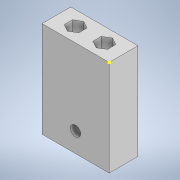
# Autodesk Inventor part: bumper piece 1
Saved by Autodesk Inventor 2022 (Build 260153000, 153)
## iProperties
Created: 2023-01-09
Part Number: bumper piece 1
Material: Generic
Document SubType Name: Modeling
Designer: s143573
Density: 1 g/cm^3
Appearance: Default
Author: s143573
Autodesk Inventor part; units mm, degrees
ref_plane "YZ Plane" through (0, 0, 0) normal (1, 0, 0) x (0, 1, 0)
ref_plane "XZ Plane" through (0, 0, 0) normal (0, 1, 0) x (-1, 0, 0)
ref_plane "XY Plane" through (0, 0, 0) normal (0, 0, 1) x (1, 0, 0)
sketch "Sketch2" plane through (0, 0, 0) normal (0, 1, 0) x (-1, 0, 0)
  line L0 (0, 0) -> (44.45, 0)
  line L1 (44.45, 0) -> (44.45, -19.05)
  line L2 (44.45, -19.05) -> (0, -19.05)
  line L3 (0, -19.05) -> (0, 0)
  dimension "d2" = 19.05
  dimension "d3" = 44.45
  constraints: 8 end point, 2 parallel, 1 horizontal, 1 perpendicular
  measures "d2" distance of L0.end L1.end
  measures "d3" distance of L1.end L2.end
extrude "Extrusion2" add sketch "Sketch2" along normal blind 63.5
sketch "Sketch6" plane through (0, 63.5, 0) normal (0, 1, 0) x (1, 0, 0)
  line L0 (-44.45, 19.05) -> (-44.45, 0) projected
  line L1 (-44.45, 9.525) -> (0, 9.525)
  line L2 (0, 0) -> (0, 19.05) projected
  line L3 (-31.8346, 15.0114) -> (-27.041, 12.3415)
  line L4 (-27.041, 12.3415) -> (-26.9563, 6.8551)
  line L5 (-26.9563, 6.8551) -> (-31.6654, 4.0386)
  line L6 (-31.6654, 4.0386) -> (-36.459, 6.7085)
  line L7 (-36.459, 6.7085) -> (-36.5437, 12.1949)
  line L8 (-36.5437, 12.1949) -> (-31.8346, 15.0114)
  line L9 (-17.5245, 12.1415) -> (-12.8464, 15.0114)
  line L10 (-12.8464, 15.0114) -> (-8.0218, 12.3949)
  line L11 (-8.0218, 12.3949) -> (-7.8755, 6.9085)
  line L12 (-7.8755, 6.9085) -> (-12.5536, 4.0386)
  line L13 (-12.5536, 4.0386) -> (-17.3782, 6.6551)
  line L14 (-17.3782, 6.6551) -> (-17.5245, 12.1415)
  point P0 (-31.75, 9.525)
  point P1 (-12.7, 9.525)
  dimension "d17" = 44.45
  dimension "d18" = 10.9728
  dimension "d19" = 10.9728
  dimension "d20" = 12.7
  dimension "d21" = 12.7
  constraints: 26 end point, 2 midpoint, 2 point on line, 26 other
  measures "d17" distance of L1.start L1.end
  measures "d18" vertical distance of L3.start L5.end
  measures "d19" vertical distance of L9.end L12.end
  measures "d20" distance of L1.start point (-31.75, 9.525)
  measures "d21" distance of L1.end point (-12.7, 9.525)
extrude "Extrusion3" cut sketch "Sketch6" against normal blind 8.382
sketch "Sketch17" plane through (0, 0, -19.05) normal (0, 0, -1) x (-1, 0, 0)
  circle A0 centre (22.225, 13.0433) radius 3.3782
  line L0 (44.45, 0) -> (44.45, 63.5) projected
  point P0 (0, 0)
  dimension "d58" = 22.225
  dimension "d59" = 6.7564
  constraints: 1 centre point
  measures "d58" distance from line of L0 A0.centre
  measures "d59" diameter of A0
extrude "Extrusion11" cut sketch "Sketch17" against normal blind 25.4
sketch "Sketch19" plane through (0, 63.5, 0) normal (0, 1, 0) x (1, 0, 0)
  point P0 (0, 0)
sketch "Sketch20" plane through (0, 63.5, 0) normal (0, 1, 0) x (1, 0, 0)
  line L0 (-7.8755, 6.9085) -> (-12.5536, 4.0386) projected
  line L1 (-12.5536, 4.0386) -> (-17.3782, 6.6551) projected
  line L2 (-17.3782, 6.6551) -> (-17.5245, 12.1415) projected
  line L3 (-17.5245, 12.1415) -> (-12.8464, 15.0114) projected
  line L4 (-12.8464, 15.0114) -> (-8.0218, 12.3949) projected
  line L5 (-8.0218, 12.3949) -> (-7.8755, 6.9085) projected
  line L6 (-17.5245, 12.1415) -> (-12.8464, 15.0114) projected
  line L7 (-17.3782, 6.6551) -> (-17.5245, 12.1415) projected
  line L8 (-12.5536, 4.0386) -> (-17.3782, 6.6551) projected
  line L9 (-7.8755, 6.9085) -> (-12.5536, 4.0386) projected
  line L10 (-8.0218, 12.3949) -> (-7.8755, 6.9085) projected
  line L11 (-12.8464, 15.0114) -> (-8.0218, 12.3949) projected
  line L12 (-26.9563, 6.8551) -> (-31.6654, 4.0386) projected
  line L13 (-27.041, 12.3415) -> (-26.9563, 6.8551) projected
  line L14 (-31.8346, 15.0114) -> (-27.041, 12.3415) projected
  line L15 (-36.5437, 12.1949) -> (-31.8346, 15.0114) projected
  line L16 (-36.459, 6.7085) -> (-36.5437, 12.1949) projected
  line L17 (-31.6654, 4.0386) -> (-36.459, 6.7085) projected
  line L18 (-7.8755, 6.9085) -> (-12.5536, 4.0386) projected
  line L19 (-12.5536, 4.0386) -> (-12.8464, 15.0114)
  line L20 (-8.0218, 12.3949) -> (-7.8755, 6.9085) projected
  line L21 (-7.9486, 9.6517) -> (-17.4514, 9.3983)
  line L22 (-17.3782, 6.6551) -> (-17.5245, 12.1415) projected
  circle A0 centre (-12.7, 9.525) radius 3.3782
  line L23 (-31.6654, 4.0386) -> (-31.8346, 15.0114)
  line L24 (-36.459, 6.7085) -> (-36.5437, 12.1949) projected
  line L25 (-36.5014, 9.4517) -> (-26.9986, 9.5983)
  line L26 (-27.041, 12.3415) -> (-26.9563, 6.8551) projected
  circle A1 centre (-31.75, 9.525) radius 3.3782
  point P0 (0, 0)
  dimension "d64" = 6.7564
  dimension "d65" = 6.7564
  constraints: 8 end point, 6 midpoint, 2 centre point, 2 point on line
  measures "d64" diameter of A0
  measures "d65" diameter of A1
extrude "Extrusion12" cut sketch "Sketch20" against normal through all contours A0 L21 L19 | L19 L21 A0 | L21 L19 A0 | L21 A0 L19 | A1 L25 L23 | L23 L25 A1 | L25 L23 A1 | L25 A1 L23
body "Solid2"
